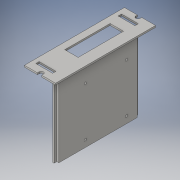
# Autodesk Inventor part: Slot
Saved by Autodesk Inventor 2016 (Build 200138000, 138)
## iProperties
Created: 2018-07-17
Part Number: Slot
Material: Generic
Document SubType Name: Modeling
Designer: Jorian Bruslind
Density: 1 g/cm^3
Appearance: Default
Author: Jorian Bruslind
Autodesk Inventor part; units mm, degrees
ref_plane "YZ Plane" through (0, 0, 0) normal (1, 0, 0) x (0, 1, 0)
ref_plane "XZ Plane" through (0, 0, 0) normal (0, 1, 0) x (-1, 0, 0)
ref_plane "XY Plane" through (0, 0, 0) normal (0, 0, 1) x (1, 0, 0)
sketch "Sketch1" plane through (0, 0, 0) normal (0, 1, 0) x (-1, 0, 0)
  line L0 (0, 0) -> (37, 0)
  line L1 (37, 0) -> (37, -119)
  line L2 (37, -119) -> (0, -119)
  line L3 (0, -119) -> (0, 0)
  dimension "d0" = 37
  dimension "d1" = 119
  constraints: 8 end point, 2 parallel, 1 horizontal, 1 perpendicular
  measures "d0" distance of L1.end L2.end
  measures "d1" distance of L0.end L1.end
extrude "Extrusion1" add sketch "Sketch1" along normal blind 2
sketch "Sketch3" plane through (0, 0, 0) normal (0, -1, 0) x (1, 0, 0)
  line L0 (0, 0) -> (-16.5, 0)
  line L1 (-37, 0) -> (0, 0) projected
  line L2 (-19, 0) -> (-19, -2)
  arc A0 (-21.5, -2) -> (-16.5, -2) centre (-19, -2) ccw
  line L3 (0, 0) -> (0, -119) projected
  line L4 (0, -119) -> (-19, -119)
  line L5 (0, -119) -> (-37, -119) projected
  line L6 (-19, -119) -> (-19, -117)
  arc A1 (-16.5, -117) -> (-21.5, -117) centre (-19, -117) ccw
  line L7 (-16.5, -117) -> (-16.5, -119)
  line L8 (-21.5, -117) -> (-21.5, -119)
  line L9 (-21.5, -119) -> (-16.5, -119)
  line L10 (-21.5, -2) -> (-21.5, 0)
  line L11 (-16.5, -2) -> (-16.5, 0)
  line L12 (-21.5, 0) -> (-16.5, 0)
  dimension "d14" = 19
  dimension "d15" = 2
  dimension "d16" = 5
  dimension "d17" = 19
  dimension "d18" = 2
  dimension "d19" = 5
  constraints: 20 end point, 6 point on line, 5 perpendicular, 4 point on circle, 2 centre point, 2 coincident, 2 horizontal, 1 parallel, 1 tangent
  measures "d14" distance of L0.start L2.start
  measures "d15" distance of L2.start L2.end
  measures "d16" diameter of A0
  measures "d17" distance of L3.end L4.end
  measures "d18" distance of L4.end L6.end
  measures "d19" diameter of A1
extrude "Extrusion3" cut sketch "Sketch3" against normal blind 2
sketch "Sketch4" plane through (0, 2, 0) normal (0, 1, 0) x (1, 0, 0)
  line L0 (0, 119) -> (0, 0) projected
  line L1 (0, 0) -> (0, 12)
  line L2 (0, 12) -> (-6, 12)
  line L3 (-32, 12) -> (-32, 105)
  line L4 (-6, 105) -> (-6, 12)
  line L5 (-11.7, 105) -> (-11.7, 108.4)
  line L6 (-11.7, 108.4) -> (-10.4, 108.4)
  line L7 (-10.4, 108.4) -> (-10.4, 105)
  line L8 (-6, 12) -> (-8, 12)
  line L9 (-8, 12) -> (-8, 105)
  line L10 (-11.7, 105) -> (-11.7, 102)
  line L11 (-11.7, 102) -> (-10.2, 102)
  line L12 (-10.2, 102) -> (-10.2, 15)
  line L13 (-32, 105) -> (-11.7, 105)
  line L14 (-10.2, 15) -> (-11.7, 15)
  line L15 (-11.7, 15) -> (-11.7, 12)
  line L16 (-11.7, 12) -> (-11.7, 8.6)
  line L17 (-11.7, 8.6) -> (-10.4, 8.6)
  line L18 (-10.4, 8.6) -> (-10.4, 12)
  line L19 (-10.4, 12) -> (-8, 12)
  line L20 (-6, 105) -> (-8, 105)
  line L21 (-8, 105) -> (-10.4, 105)
  line L22 (-32, 12) -> (-11.7, 12)
  point P0 (-19, 2)
  dimension "d59" = 12
  dimension "d60" = 6
  dimension "d61" = 26
  dimension "d62" = 93
  dimension "d73" = 2
  dimension "d121" = 2
  dimension "d122" = 93
  dimension "d125" = 20.3
  dimension "d126" = 20.3
  dimension "d127" = 3.4
  dimension "d128" = 3.4
  dimension "d129" = 87
  dimension "d130" = 2.2
  dimension "d154" = 1.3
  dimension "d155" = 1.3
  dimension "d156" = 4.4
  dimension "d157" = 4.4
  dimension "d158" = 1.5
  dimension "d159" = 1.5
  constraints: 44 end point, 6 horizontal, 4 perpendicular, 2 parallel, 2 point on line, 1 collinear, 1 vertical
  measures "d59" distance of L0.end L1.end
  measures "d60" distance of L1.end L2.end
  measures "d61" distance of L3.end L4.start
  measures "d62" distance of L3.start L3.end
  measures "d73" distance of L2.end L8.end
  measures "d121" distance of L4.start L9.end
  measures "d122" distance of L4.start L2.end
  measures "d125" distance of L3.start L15.end
  measures "d126" distance of L3.end L5.start
  measures "d127" distance of L15.end L16.end
  measures "d128" distance of L5.start L5.end
  measures "d129" distance of L11.end L12.end
  measures "d130" distance between parallel lines of L9 L12
  measures "d154" distance of L5.end L6.end
  measures "d155" distance of L16.end L17.end
  measures "d156" distance between parallel lines of L18 L4
  measures "d157" distance between parallel lines of L7 L4
  measures "d158" distance of L10.end L11.end
  measures "d159" distance of L12.end L14.end
extrude "Extrusion7" add sketch "Sketch4" against normal blind 92 contours L15 L14 L12 L11 L10 L5 L6 L7 L21 L9 L19 L18 L17 L16
sketch "Sketch6" plane through (-10.2, -90, -102) normal (-1, 0, 0) x (0, 0, 1)
  line L0 (102, 92) -> (-17, 92) projected
  line L1 (-6.4, 92) -> (58.6, 92)
  line L2 (58.6, 92) -> (58.6, 66.128)
  circle A0 centre (58.6, 66.128) radius 1.375
  line L3 (-6.4, 90) -> (-6.4, 0) projected
  line L4 (58.6, 66.128) -> (58.6, 8.128)
  circle A1 centre (58.6, 8.128) radius 1.375
  line L5 (58.6, 8.128) -> (9.6, 8.128)
  circle A2 centre (9.6, 8.128) radius 1.375
  line L6 (9.6, 8.128) -> (9.6, 66.128)
  circle A3 centre (9.6, 66.128) radius 1.375
  point P0 (102, 90)
  dimension "d80" = 65
  dimension "d81" = 25.872
  dimension "d82" = 2.75
  dimension "d83" = 65
  dimension "d87" = 58
  dimension "d88" = 2.75
  dimension "d89" = 49
  dimension "d90" = 2.75
  dimension "d91" = 2.75
  constraints: 10 end point, 4 centre point, 4 coincident, 2 point on line, 2 vertical, 1 horizontal, 1 perpendicular
  measures "d80" distance of L1.start L1.end
  measures "d81" distance of L1.end L2.end
  measures "d82" diameter of A0
  measures "d83" distance between parallel lines of L3 L2
  measures "d87" distance of L4.start L4.end
  measures "d88" diameter of A1
  measures "d89" distance of L5.start L5.end
  measures "d90" diameter of A2
  measures "d91" diameter of A3
extrude "Extrusion8" cut sketch "Sketch6" against normal blind 2.2
sketch "Sketch7" plane through (0, 0, 0) normal (0, -1, 0) x (1, 0, 0)
  line L0 (-10.2, -102) -> (-10.2, -15) projected
  line L1 (-10.2, -102) -> (-10.2, -40)
  line L2 (-10.2, -40) -> (-13.1, -40)
  line L3 (-13.1, -40) -> (-29.1, -40)
  line L4 (-29.1, -40) -> (-29.1, -94)
  line L5 (-29.1, -94) -> (-13.1, -94)
  line L6 (-13.1, -94) -> (-13.1, -40)
  point P0 (0, 0)
  point P1 (-10, -12)
  point P2 (-10.2, -15)
  dimension "d94" = 62
  dimension "d95" = 2.9
  dimension "d96" = 16
  dimension "d97" = 54
  constraints: 12 end point, 2 horizontal, 2 parallel, 1 perpendicular, 2 other
  measures "d94" distance of L1.start L1.end
  measures "d95" distance of L1.end L2.end
  measures "d96" distance of L5.end L4.end
  measures "d97" distance of L4.end L3.end
extrude "Extrusion9" cut sketch "Sketch7" against normal blind 2
sketch "Sketch9" plane through (0, 2, 0) normal (0, 1, 0) x (1, 0, 0)
  line L0 (0, 0) -> (0, 119) projected
  arc A0 (-16.5, 2) -> (-21.5, 2) centre (-19, 2) ccw projected
  line L1 (-19, 2) -> (-19, 8.5)
  line L2 (-37, 0) -> (-37, 119) projected
  line L3 (-37, 8.5) -> (-32, 8.5)
  line L4 (-32, 8.5) -> (-12, 8.5)
  line L5 (-12, 8.5) -> (-12, 12.5)
  line L6 (-12, 12.5) -> (-32, 12.5)
  line L7 (-32, 12.5) -> (-32, 8.5)
  line L8 (-37, 0) -> (-21.5, 0) projected
  arc A1 (-21.5, 117) -> (-16.5, 117) centre (-19, 117) ccw projected
  line L9 (-19, 117) -> (-19, 110.5)
  line L10 (-37, 110.5) -> (-32, 110.5)
  line L11 (-32, 110.5) -> (-12, 110.5)
  line L12 (-12, 110.5) -> (-12, 106.5)
  line L13 (-12, 106.5) -> (-32, 106.5)
  line L14 (-32, 106.5) -> (-32, 110.5)
  line L15 (-21.5, 119) -> (-37, 119) projected
  dimension "d142" = 6.5
  dimension "d143" = 5
  dimension "d144" = 20
  dimension "d145" = 4
  dimension "d146" = 12.5
  dimension "d147" = 6.5
  dimension "d148" = 5
  dimension "d149" = 20
  dimension "d150" = 4
  dimension "d151" = 12.5
  constraints: 24 end point, 5 parallel, 4 horizontal, 2 perpendicular, 2 point on line, 1 vertical
  measures "d142" distance of L1.start L1.end
  measures "d143" distance of L3.start L3.end
  measures "d144" distance of L6.end L5.end
  measures "d145" distance of L5.end L4.end
  measures "d146" distance between parallel lines of L8 L6
  measures "d147" distance of L9.start L9.end
  measures "d148" distance of L10.start L10.end
  measures "d149" distance of L12.end L13.end
  measures "d150" distance of L11.end L12.end
  measures "d151" distance between parallel lines of L15 L13
extrude "Extrusion11" cut sketch "Sketch9" against normal blind 2
body "Solid1"
